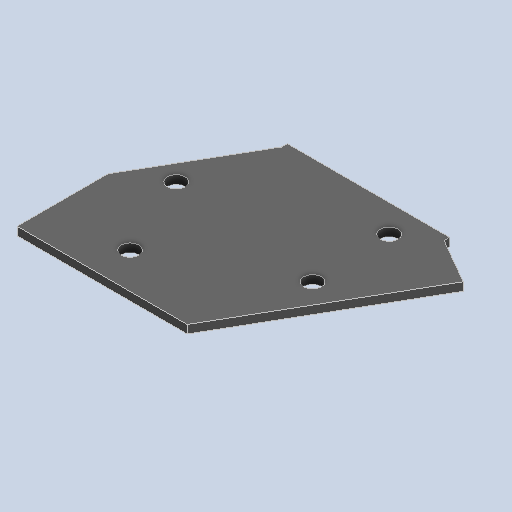
# Autodesk Inventor part: rail_cover_upper
Saved by Autodesk Inventor 2024.1 (Build 281209000, 209)
## iProperties
Created: 2025-01-17
Part Number: rail_cover_upper
Material: 一般
Document SubType Name: Modeling
Designer: hibik
Density: 1 g/cm^3
Appearance: 既定
Author: hibik
Autodesk Inventor part; units mm, degrees
ref_plane "YZ Plane" through (0, 0, 0) normal (1, 0, 0) x (0, 1, 0)
ref_plane "XZ Plane" through (0, 0, 0) normal (0, 1, 0) x (-1, 0, 0)
sketch "スケッチ1" plane through (0, 0, 0) normal (0, 1, 0) x (-1, 0, 0)
  line L0 (0, 0) -> (30, 0)
  line L1 (30, 0) -> (30, -135.2775)
  line L2 (30, -135.2775) -> (-78.1025, -135.2775)
  line L3 (-78.1025, -135.2775) -> (0, 0)
  dimension "d0" = 30
  dimension "d1" = 60
  constraints: 8 end point, 2 horizontal, 1 vertical
  measures "d0" distance of L0.start L0.end
  measures "d1" angle of L0 L3
extrude "押し出し1" add sketch "スケッチ1" along normal blind 1.5
sketch "スケッチ2" plane through (0, 1.5, 0) normal (0, 1, 0) x (1, 0, 0)
  line L0 (-25, 8) -> (-25, 1.5) projected
  line L1 (-21.9199, 13.3349) -> (-25, 8) projected
  line L2 (-30, 18) -> (-21.9199, 13.3349) projected
  line L3 (-24.2265, 28) -> (-30, 18) projected
  line L4 (0, 28) -> (-24.2265, 28) projected
  line L5 (10.9697, 38) -> (0, 38) projected
  line L6 (13.5677, 36.5) -> (10.9697, 38) projected
  line L7 (11.0677, 32.1699) -> (13.5677, 36.5) projected
  line L8 (16.6969, 28.9199) -> (11.0677, 32.1699) projected
  line L9 (7.3612, 12.75) -> (16.6969, 28.9199) projected
  line L10 (0, 17) -> (7.3612, 12.75) projected
  line L11 (-12, 17) -> (0, 17) projected
  line L12 (-12, 8) -> (-12, 17) projected
  line L13 (-5, 8) -> (-12, 8) projected
  line L14 (-5, 1.5) -> (-5, 8) projected
  line L15 (-25, 1.5) -> (-5, 1.5) projected
  line L16 (78.1025, 135.2775) -> (-30, 135.2775) projected
  line L17 (-30, 135.2775) -> (-30, 0) projected
  line L18 (-30, 0) -> (0, 0) projected
  line L19 (0, 0) -> (78.1025, 135.2775) projected
  line L20 (-24.2265, 28) -> (-18.453, 38)
  line L21 (-18.453, 38) -> (5, 38)
  line L22 (13.5677, 36.5) -> (19.1969, 33.25)
  line L23 (0, 28) -> (0, 38) projected
  circle A0 centre (5, 34) radius 2.5 projected
  circle A1 centre (5.5311, 19.5801) radius 1.35 projected
  circle A2 centre (-16, 8) radius 1.35 projected
  circle A3 centre (-22.5359, 22.9282) radius 1.35 projected
  circle A4 centre (-6, 23) radius 1.35 projected
  line L24 (-30, 1.5) -> (-25, 1.5)
  line L25 (-5, 1.5) -> (0.866, 1.5)
  point P0 (0, 36.5)
  point P1 (5, 36.5)
  constraints: 10 end point, 4 point on line, 2 horizontal, 1 collinear, 1 perpendicular, 1 vertical alignment
extrude "押し出し2" cut sketch "スケッチ2" against normal through all contours L15 L25 L19 L18 L17 L24 | L17 L16 L19 L22 L6 L5 L21 L20 L3
sketch "スケッチ3" plane through (0, 1.5, 0) normal (0, 1, 0) x (1, 0, 0)
  line L0 (-18.453, 38) -> (10.9697, 38) projected
  line L1 (5, 36.5) -> (-17, 36.5) projected
  line L2 (10.9697, 39) -> (-18.453, 39)
  line L3 (-18.453, 39) -> (-18.453, 35.5)
  line L4 (-18.453, 35.5) -> (10.9697, 35.5)
  line L5 (10.9697, 35.5) -> (10.9697, 39)
  line L6 (5, 36.5) -> (10.9697, 36.5)
  line L7 (-17, 36.5) -> (-18.453, 36.5)
  point P0 (0, 0)
  dimension "d6" = 1
  dimension "d7" = 1
  constraints: 12 end point, 5 point on line, 2 parallel, 2 perpendicular, 1 horizontal
  measures "d6" distance between parallel lines of L2 L0
  measures "d7" distance between parallel lines of L4 L1
extrude "押し出し3" add sketch "スケッチ3" against normal blind 3.5 contours L3 L2 L5 L0 | L7 L1 L6 L5 L4 L3
sketch "スケッチ4" plane through (0, 1.5, 0) normal (0, 1, 0) x (1, 0, 0)
  circle A0 centre (-16, 8) radius 1.6
  circle A1 centre (-22.5359, 22.9282) radius 1.6
  circle A2 centre (5.5311, 19.5801) radius 1.6
  circle A3 centre (5, 34) radius 1.6
  line L0 (0, 36.5) -> (0, 17) projected
  line L1 (-12, 8) -> (-12, 28) projected
  line L2 (-18.453, 38) -> (-30, 18) projected
  line L3 (-30, 18) -> (-21.9199, 13.3349) projected
  line L4 (0, 17) -> (7.3612, 12.75) projected
  line L5 (0.866, 1.5) -> (19.1969, 33.25) projected
  line L6 (10.9697, 39) -> (-18.453, 39) projected
  circle A4 centre (5, 34) radius 2.5 projected
  point P0 (0, 0)
  point P1 (16.6969, 28.9199)
  dimension "d10" = 3.2
  dimension "d11" = 3.2
  dimension "d12" = 3.2
  dimension "d13" = 3.2
  dimension "d14" = 4
  dimension "d15" = 4
  dimension "d16" = 8
  dimension "d17" = 5
  dimension "d18" = 5
  constraints: 4 centre point, 1 concentric, 1 horizontal alignment
  measures "d10" diameter of A0
  measures "d11" diameter of A1
  measures "d12" diameter of A2
  measures "d13" diameter of A3
  measures "d14" distance from line of L1 A0.centre
  measures "d15" distance from line of L2 A1.centre
  measures "d16" distance from line of L3 A1.centre
  measures "d17" distance from line of L4 A2.centre
  measures "d18" distance from line of L5 A2.centre
extrude "押し出し4" cut sketch "スケッチ4" against normal through all contours A0 | A1 | A2 | A3
sketch "スケッチ5" plane through (0, -2, 0) normal (0, -1, 0) x (1, 0, 0)
  line L0 (10.9697, -39) -> (3.9697, -39)
  line L1 (3.9697, -39) -> (3.9697, -35.5)
  line L2 (3.9697, -35.5) -> (10.9697, -35.5)
  line L3 (10.9697, -35.5) -> (10.9697, -39)
  line L4 (10.9697, -35.5) -> (5.5568, -35.5) projected
  point P0 (0, 0)
  dimension "d23" = 7
  constraints: 8 end point, 2 parallel, 1 collinear, 1 horizontal, 1 perpendicular
  measures "d23" distance between parallel lines of L3 L1
extrude "押し出し5" cut sketch "スケッチ5" against normal up to surface (2 mm away)
sketch "スケッチ6" plane through (0, -2, 0) normal (0, -1, 0) x (1, 0, 0)
  line L0 (-18.453, -36.5) -> (3.9697, -36.5) projected
  line L1 (3.9697, -36.5) -> (3.9697, -35.5) projected
  line L2 (3.9697, -35.5) -> (-18.453, -35.5) projected
  line L3 (-1.0303, -36.5) -> (-1.0303, -35.5)
  point P0 (0, 0)
  dimension "d26" = 5
  constraints: 2 end point, 2 point on line, 1 perpendicular
  measures "d26" distance between parallel lines of L1 L3
ref_plane "作業平面1" through (0, 0, -38) normal (0, 1, 0) x (0, 0, 1)
extrude "押し出し6" cut sketch "スケッチ6" against normal up to surface (2 mm away)
